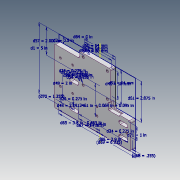
# Autodesk Inventor part: J005167
Saved by Autodesk Inventor 2015 SP1 (Build 190203100, 203)
## iProperties
Created: 2015-04-09
Material: ALUMINUM, 6061-T651
Vendor: HHMI: JRC - ID&F
Document SubType Name: Modeling
Designer: ARNOLDJ
Density: 2.7 g/cm^3
Appearance: Metal-AL-6061 (Machined)
Part Number: J005167
Description: MBS POSITIONER BASE PLATE
Project: P-201804
RuleStatus: InUse
AfterDocSave0: file://Part Number Cleaner
LAB/DEPT: SVOBODA (LAB)
REQUESTING SCIENTIST: SOFRONIEW, NICK
SURFACE ROUGHNESS: 63 Ra
DESIGN DEPARTMENT: HHMI: JRC - ID&F
SPECIAL FINISH: ANODIZE PER MIL-A-8625F, TYPE II, CLASS 2 (BLACK)
ALTERED ITEM PART NUMBER: N/A
ALTERED ITEM VENDOR: N/A
ALTERED ITEM DESCRIPTION: N/A
Revision Number: A
Autodesk Inventor part; units mm, degrees
ref_plane "YZ Plane" through (0, 0, 0) normal (1, 0, 0) x (0, 1, 0)
ref_plane "XZ Plane" through (0, 0, 0) normal (0, 1, 0) x (-1, 0, 0)
ref_plane "XY Plane" through (0, 0, 0) normal (0, 0, 1) x (1, 0, 0)
sketch "Sketch1" plane through (0, 0, 0) normal (0, 0, 1) x (1, 0, 0)
  line L0 (73.66, -76.2) -> (-84.709, -76.2)
  line L1 (-84.709, -76.2) -> (-84.709, 50.8)
  line L2 (-84.709, 50.8) -> (73.66, 50.8)
  line L3 (73.66, 50.8) -> (73.66, -76.2)
  line L4 (-84.709, 50.8) -> (-32, 50.8)
  line L5 (-32, 50.8) -> (-32, 38.1)
  line L6 (-32, 38.1) -> (-84.709, 38.1)
  line L7 (-84.709, 38.1) -> (-84.709, 50.8)
  line L8 (73.66, 50.8) -> (32, 50.8)
  line L9 (32, 50.8) -> (32, -22.225)
  line L10 (32, -22.225) -> (73.66, -22.225)
  line L11 (73.66, -22.225) -> (73.66, 50.8)
  line L12 (-34.4202, -12.5158) -> (-52.8352, -12.5158)
  line L13 (-52.8352, -12.5158) -> (-52.8352, -5.5308)
  line L14 (-52.8352, -5.5308) -> (-34.4202, -5.5308)
  line L15 (-34.4202, -5.5308) -> (-34.4202, -12.5158)
  line L16 (-34.4202, -12.5158) -> (-52.8352, -5.5308) construction
  line L17 (-52.8352, -12.5158) -> (-34.4202, -5.5308) construction
  line L18 (-34.4202, -63.3158) -> (-52.8352, -63.3158)
  line L19 (-52.8352, -63.3158) -> (-52.8352, -56.3308)
  line L20 (-52.8352, -56.3308) -> (-34.4202, -56.3308)
  line L21 (-34.4202, -56.3308) -> (-34.4202, -63.3158)
  line L22 (-34.4202, -63.3158) -> (-52.8352, -56.3308) construction
  line L23 (-52.8352, -63.3158) -> (-34.4202, -56.3308) construction
  line L24 (48.7648, -63.3158) -> (67.1798, -63.3158)
  line L25 (67.1798, -63.3158) -> (67.1798, -56.3308)
  line L26 (67.1798, -56.3308) -> (48.7648, -56.3308)
  line L27 (48.7648, -56.3308) -> (48.7648, -63.3158)
  line L28 (48.7648, -63.3158) -> (67.1798, -56.3308) construction
  line L29 (67.1798, -63.3158) -> (48.7648, -56.3308) construction
  line L30 (-43.6277, -59.8233) -> (-43.6277, -9.0233) construction
  line L31 (-43.6277, -59.8233) -> (-43.6277, -56.3308) construction
  line L32 (-25, 43.8) -> (25, 43.8) construction
  line L33 (25, 43.8) -> (25, -6.2) construction
  line L34 (25, -6.2) -> (-25, -6.2) construction
  line L35 (-25, -6.2) -> (-25, 43.8) construction
  line L36 (-25, 18.8) -> (25, 18.8) construction
  line L37 (57.9723, -59.8233) -> (-43.6277, -59.8233) construction
  line L38 (0, 43.8) -> (0, -6.2) construction
  line L39 (32, -13.2) -> (-32, -13.2) construction
  line L40 (-32, -13.2) -> (-32, 50.8) construction
  line L41 (-32, 50.8) -> (32, 50.8) construction
  line L42 (32, 50.8) -> (32, -13.2) construction
  line L43 (32, -13.2) -> (-32, 50.8) construction
  line L44 (-32, -13.2) -> (32, 50.8) construction
  circle A0 centre (-37.6333, -9.0233) radius 3.0299 construction
  circle A1 centre (-43.6277, -9.0233) radius 2.9972 construction
  circle A2 centre (-37.6333, -9.0233) radius 4.7625 construction
  line L45 (0, 76.2) -> (0, -101.6) projected
  line L46 (57.9723, -59.8233) -> (57.9723, -34.4233) construction
  line L47 (67.1798, -30.9308) -> (48.7648, -30.9308)
  line L48 (48.7648, -30.9308) -> (48.7648, -37.9158)
  line L49 (48.7648, -37.9158) -> (67.1798, -37.9158)
  line L50 (67.1798, -37.9158) -> (67.1798, -30.9308)
  line L51 (67.1798, -30.9308) -> (48.7648, -37.9158) construction
  line L52 (48.7648, -30.9308) -> (67.1798, -37.9158) construction
  point P0 (0, 0)
  point P1 (0, 0)
  point P2 (0, 0)
  point P3 (0, 18.8)
  dimension "d1" = 127
  dimension "d2" = 12.7
  dimension "d24" = 6.985
  dimension "d25" = 18.415
  dimension "d26" = 6.985
  dimension "d34" = 6.985
  dimension "d40" = 50
  dimension "d41" = 50
  dimension "d45" = 101.6
  dimension "d48" = 59.8233
  dimension "d49" = 50.8
  dimension "d50" = 64
  dimension "d51" = 64
  dimension "d52" = 0
  dimension "d53" = 5.9944
  dimension "d54" = 5.9944
  dimension "d57" = 50.8
  dimension "d60" = 9.525
  dimension "d61" = 73.025
  dimension "d63" = 64
  dimension "d64" = 0
  dimension "d65" = 84.709
  dimension "d66" = 73.66
  dimension "d67" = 43.6277
  dimension "d68" = 6.4802
  dimension "d69" = 158.369
  dimension "d70" = 31.8738
  dimension "d71" = 25.4
  constraints: 104 end point, 22 parallel, 14 midpoint, 9 horizontal, 9 perpendicular, 6 coincident, 3 centre point, 2 vertical, 1 point on line
  measures "d1" distance of L0.end L1.end
  measures "d2" distance of L4.end L5.end
  measures "d24" distance of L12.end L13.end
  measures "d25" distance of L13.end L14.end
  measures "d26" distance of L18.end L19.end
  measures "d34" distance of L26.end L24.start
  measures "d40" distance of L32.start L32.end
  measures "d41" distance of L32.end L33.end
  measures "d45" distance of L37.start L37.end
  measures "d48" distance from line of point (0, 0) L37
  measures "d49" distance of L30.start L30.end
  measures "d50" distance of L40.end L41.end
  measures "d51" distance of L39.end L40.end
  measures "d52" distance between parallel lines of L2 L41
  measures "d53" diameter of A1
  measures "d54" distance of L30.end A0.centre
  measures "d57" distance from line of point (0, 0) L4
  measures "d60" diameter of A2
  measures "d61" distance between parallel lines of L10 L8
  measures "d63" distance between parallel lines of L5 L9
  measures "d64" distance between parallel lines of L40 L5
  measures "d65" distance between parallel lines of L1 L45
  measures "d66" distance between parallel lines of L45 L3
  measures "d67" distance between parallel lines of L45 L30
  measures "d68" distance between parallel lines of L3 L25
  measures "d69" distance between parallel lines of L3 L1
  measures "d70" distance between parallel lines of L1 L19
  measures "d71" distance of L37.start L46.end
extrude "Extrusion1" add sketch "Sketch1" along normal blind 9.525 contours L0 L45 L2 L9 L10 L3 | L0 L1 L6 L5 L2 L45 | L12 L13 L14 L15 | L18 L19 L20 L21 | L27 L26 L25 L24 | L50 L49 L48 L47
hole "Hole1" at (-25, 43.8, 0) at (25, 43.8, 0) at (25, -6.2, 0) at (-25, -6.2, 0) direction (0, 0, 1) diameter 4.9276 end through all
extrude "Extrusion2" cut sketch "Sketch1" along normal up to next contours L12 L13 L14 L15 | L18 L19 L20 L21 | L27 L26 L25 L24 | L50 L49 L48 L47
sketch "Sketch3" plane through (0, 0, 9.525) normal (0, 0, 1) x (1, 0, 0)
  line L0 (73.66, -22.225) -> (32, -22.225) projected
  line L1 (32, -22.225) -> (32, 50.8) projected
  line L2 (27.6058, -24.9428) -> (50.6944, -24.9428)
  line L3 (50.6944, -24.9428) -> (50.6944, -9.9084)
  line L4 (50.6944, -9.9084) -> (27.6058, -9.9084)
  line L5 (27.6058, -9.9084) -> (27.6058, -24.9428)
  point P0 (0, 0)
  dimension "d99" = 23.0886
  dimension "d100" = 2.7178
  dimension "d101" = 4.3942
  constraints: 8 end point, 2 parallel, 1 horizontal, 1 perpendicular
  measures "d99" distance of L3.end L4.end
  measures "d100" distance between parallel lines of L0 L2
  measures "d101" distance between parallel lines of L5 L1
extrude "Extrusion4" cut sketch "Sketch3" against normal blind 6.731
fillet "Fillet1" radius 3.175 8 edges at (-32, 38.1, 4.7625) (-32, 50.8, 4.7625) (32, 50.8, 4.7625) (73.66, -22.225, 4.7625) (-84.709, 38.1, 4.7625) (-84.709, -76.2, 4.7625) (73.66, -76.2, 4.7625) (32, -22.225, 1.397)
fillet "Fillet2" radius 3.175 16 edges at (-52.8352, -63.3158, 4.7625) (-52.8352, -12.5158, 4.7625) (-52.8352, -56.3308, 4.7625) (-52.8352, -5.5308, 4.7625) (48.7648, -63.3158, 4.7625) (48.7648, -56.3308, 4.7625) (67.1798, -56.3308, 4.7625) (67.1798, -63.3158, 4.7625) (-34.4202, -5.5308, 4.7625) (-34.4202, -12.5158, 4.7625) (-34.4202, -56.3308, 4.7625) (-34.4202, -63.3158, 4.7625) (48.7648, -30.9308, 4.7625) (48.7648, -37.9158, 4.7625) (67.1798, -30.9308, 4.7625) (67.1798, -37.9158, 4.7625)
sketch "Sketch2" plane through (0, 0, 0) normal (0, 0, 1) x (1, 0, 0)
  line L0 (-72.009, 18.796) -> (-46.609, 18.796) construction
  line L1 (-46.609, 18.796) -> (-46.609, -32.004) construction
  line L2 (-46.609, -32.004) -> (-72.009, -32.004) construction
  line L3 (-72.009, -32.004) -> (-72.009, 18.796) construction
  line L4 (-35.175, 38.1) -> (-81.534, 38.1) construction
  line L5 (-84.709, 34.925) -> (-84.709, -73.025) construction
  line L6 (-52.8352, -9.3408) -> (-52.8352, -8.7058) construction
  line L7 (-52.8352, -9.0233) -> (-63.8216, -9.0233) construction
  point P0 (0, 0)
  dimension "d73" = 25.4
  dimension "d74" = 50.8
  dimension "d75" = 19.304
  dimension "d76" = 12.7
  dimension "d77" = 47.1232
  constraints: 10 end point, 4 coincident, 2 horizontal, 2 parallel, 1 midpoint, 1 perpendicular
  measures "d73" distance of L0.start L0.end
  measures "d74" distance of L2.end L0.start
  measures "d75" distance between parallel lines of L0 L4
  measures "d76" distance between parallel lines of L5 L3
  measures "d77" distance between parallel lines of L4 L7
hole "Hole2" at (-72.009, 18.796, 0) at (-46.609, 18.796, 0) at (-46.609, -32.004, 0) at (-72.009, -32.004, 0) direction (0, 0, 1) diameter 4.1402 end through all
fillet "Fillet5" radius 1.651 4 edges at (32, -9.9084, 6.1595) (27.6058, -9.9084, 6.1595) (27.6058, -24.9428, 6.1595) (50.6944, -24.9428, 6.1595)
sketch "Sketch4" plane through (0, 0, 9.525) normal (0, 0, 1) x (1, 0, 0)
  line L0 (57.9723, -34.4233) -> (57.9723, -59.8233) construction
  line L1 (57.9723, -47.1233) -> (65.2526, -47.1233) construction
  line L2 (73.66, -73.025) -> (73.66, -25.4) construction
  point P0 (0, 0)
  point P1 (3.6576, -47.1233)
  point P2 (3.6576, -30.6133)
  dimension "d107" = 8.4074
  dimension "d115" = 61.595
  dimension "d116" = 16.51
  constraints: 4 end point, 1 coincident, 1 horizontal, 1 midpoint, 1 point on line, 1 vertical, 1 vertical alignment
  measures "d107" distance from line of L2 L1.end
  measures "d115" distance of L1.end point (3.658, -47.123)
  measures "d116" distance of point (3.658, -47.123) point (3.658, -30.613)
hole "Hole3" at (65.2526, -47.1233, 9.525) at (3.6576, -47.1233, 9.525) at (3.6576, -30.6133, 9.525) direction (0, 0, -1) diameter 4.1402 end through all
body "Solid1"
